Autodesk Inventor part; units mm, degrees
(part 2 of 2)
sketch "Sketch10" plane through (0, 4.7752, 0) normal (0, 1, 0) x (1, 0, 0)
  line L0 (-254, 76.2) -> (-431.8, 76.2)
  line L1 (-431.8, 76.2) -> (-431.8, 266.7)
  line L2 (-431.8, 266.7) -> (-254, 266.7)
  line L3 (-254, 266.7) -> (-254, 76.2)
  line L4 (-254, 76.2) -> (-431.8, 266.7) construction
  line L5 (-431.8, 76.2) -> (-254, 266.7) construction
  line L6 (-511.175, 514.35) -> (-174.625, 514.35) projected
  line L7 (-685.8, 3.175) -> (-685.8, 339.725) projected
  line L8 (-342.9, 171.45) -> (-317.5, 171.45) construction
  line L9 (-342.9, 171.45) -> (-393.7, 171.45) construction
  line L10 (-393.7, 158.75) -> (-342.9, 158.75)
  line L11 (-393.7, 184.15) -> (-342.9, 184.15)
  line L12 (-317.5, 184.15) -> (-342.9, 184.15)
  line L13 (-320.675, 184.15) -> (-390.525, 184.15)
  line L14 (-320.675, 158.75) -> (-342.9, 158.75)
  line L15 (-342.9, 158.75) -> (-390.525, 158.75)
  line L16 (-317.5, 171.45) -> (-279.4, 171.45)
  line L17 (-281.6451, 173.6951) -> (-312.0799, 204.1299)
  line L18 (-279.4, 171.45) -> (-207.558, 171.45) construction
  line L19 (-281.6451, 169.2049) -> (-312.0799, 138.7701)
  line L20 (-279.4, 171.45) -> (-207.558, 171.45) construction
  line L21 (-317.5, 155.575) -> (-317.5, 141.0151)
  line L22 (-317.5, 187.325) -> (-317.5, 201.8849)
  line L23 (-393.7, 180.975) -> (-393.7, 161.925)
  arc A0 (-390.525, 184.15) -> (-393.7, 180.975) centre (-390.525, 180.975) ccw
  arc A1 (-320.675, 184.15) -> (-317.5, 187.325) centre (-320.675, 187.325) ccw
  arc A2 (-312.0799, 204.1299) -> (-317.5, 201.8849) centre (-314.325, 201.8849) ccw
  arc A3 (-281.6451, 169.2049) -> (-281.6451, 173.6951) centre (-283.8901, 171.45) ccw
  arc A4 (-317.5, 141.0151) -> (-312.0799, 138.7701) centre (-314.325, 141.0151) ccw
  arc A5 (-317.5, 155.575) -> (-320.675, 158.75) centre (-320.675, 155.575) ccw
  arc A6 (-393.7, 161.925) -> (-390.525, 158.75) centre (-390.525, 161.925) ccw
  point P0 (0, 0)
  point P1 (-317.5, 209.55)
  dimension "d260" = 342.9
  dimension "d261" = 342.9
  dimension "d262" = 190.5
  dimension "d263" = 177.8
  dimension "d264" = 25.4
  dimension "d265" = 50.8
  dimension "d266" = 12.7
  dimension "d267" = 12.7
  dimension "d268" = 12.7
  dimension "d269" = 12.7
  dimension "d270" = 38.1
  dimension "d271" = 135
  dimension "d272" = 135
  dimension "d273" = 3.175
  dimension "d274" = 3.175
  constraints: 44 end point, 14 point on circle, 14 tangent, 7 centre point, 7 point on line, 6 horizontal, 5 equal radius, 2 midpoint, 2 parallel, 2 perpendicular, 1 vertical, 2 other
  measures "d260" distance from line of L6 L8.start
  measures "d261" distance from line of L7 L8.start
  measures "d262" distance of L0.end L1.end
  measures "d263" distance of L1.end L2.end
  measures "d264" distance of L8.start L8.end
  measures "d265" distance of L8.start L9.end
  measures "d266" distance between parallel lines of L9 L10
  measures "d267" distance between parallel lines of L9 L11
  measures "d268" distance between parallel lines of L8 L12
  measures "d269" distance between parallel lines of L8 L14
  measures "d270" distance of L8.end L16.end
  measures "d271" angle of L18 L17
  measures "d272" angle of L19 L20
  measures "d273" radius of A0
  measures "d274" radius of A2
extrude "Extrusion9" cut sketch "Sketch10" against normal through all contours A6 L23 A0 L11 L12 A1 L22 A2 L17 A3 L19 A4 L21 A5 L14 L10
ref_plane "Work Plane1" through (-342.9, 0, -3.175) normal (1, 0, 0) x (0, 0, -1)
extrude "Extrusion10" cut sketch "Sketch9" against normal through all
mirror "Mirror2" about plane through (-342.9, 0, -3.175) normal (1, 0, 0) of "Extrusion10"
equation "\"d21\" = d22"
equation "\"d22\" = d19"
equation "\"d51\" = d50"
body "Solid1"
